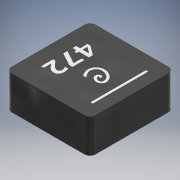
# Autodesk Inventor part: Inductor_7575
Saved by Autodesk Inventor 2018 (Build 220112000, 112)
## iProperties
Created: 2018-09-29
Part Number: Inductor_7575
Material: Steel, Carbon
Document SubType Name: Modeling
Designer: Bradley
Density: 4.9816 g/cm^3
Appearance: Fine Textured - Black
Mass: 0.85 g
Surface Area: 2.02842 cm^2
Volume: 0.170628 cm^3
Author: Bradley
Autodesk Inventor part; units mm, degrees
ref_plane "YZ Plane" through (0, 0, 0) normal (1, 0, 0) x (0, 1, 0)
ref_plane "XZ Plane" through (0, 0, 0) normal (0, 1, 0) x (-1, 0, 0)
ref_plane "XY Plane" through (0, 0, 0) normal (0, 0, 1) x (1, 0, 0)
sketch "Sketch1" plane through (0, 0, 0) normal (0, 0, 1) x (1, 0, 0)
  line L0 (3.25, -3.75) -> (-3.25, -3.75)
  line L1 (-3.75, -3.25) -> (-3.75, 3.25)
  line L2 (-3.25, 3.75) -> (3.25, 3.75)
  line L3 (3.75, 3.25) -> (3.75, -3.25)
  line L4 (3.75, -3.75) -> (-3.75, 3.75) construction
  line L5 (-3.75, -3.75) -> (3.75, 3.75) construction
  arc A0 (-3.25, 3.75) -> (-3.75, 3.25) centre (-3.25, 3.25) ccw
  arc A1 (-3.75, -3.25) -> (-3.25, -3.75) centre (-3.25, -3.25) ccw
  arc A2 (3.25, -3.75) -> (3.75, -3.25) centre (3.25, -3.25) ccw
  arc A3 (3.75, 3.25) -> (3.25, 3.75) centre (3.25, 3.25) ccw
  point P0 (0, 0)
  dimension "d0" = 7.5
  dimension "d1" = 0.5
  constraints: 12 end point, 8 point on circle, 8 point on line, 8 tangent, 4 centre point, 3 equal radius, 2 midpoint, 2 parallel, 2 perpendicular, 1 horizontal
  measures "d0" distance of L4.end L5.end
  measures "d1" radius of A0
extrude "Extrusion1" add sketch "Sketch1" along normal mid plane 3.02
sketch "Sketch2" plane through (0, 0, -1.51) normal (0, 0, -1) x (-1, 0, 0)
  line L0 (2.96, -3) -> (1.56, -3)
  line L1 (1.56, -3) -> (1.56, 3)
  line L2 (1.56, 3) -> (2.96, 3)
  line L3 (2.96, 3) -> (2.96, -3)
  line L4 (-1.56, -3) -> (-2.96, -3)
  line L5 (-2.96, -3) -> (-2.96, 3)
  line L6 (-2.96, 3) -> (-1.56, 3)
  line L7 (-1.56, 3) -> (-1.56, -3)
  line L8 (0, -3) -> (0, 3) construction
  point P0 (0, 0)
  point P1 (0, 0)
  dimension "d4" = 1.4
  dimension "d5" = 6
  dimension "d6" = 3.12
  constraints: 18 end point, 4 parallel, 4 point on line, 2 horizontal, 2 perpendicular, 1 coincident, 1 midpoint, 1 vertical, 2 other
  measures "d4" distance of L0.start L0.end
  measures "d5" distance of L2.end L0.start
  measures "d6" distance between parallel lines of L7 L1
extrude "Extrusion2" add sketch "Sketch2" along normal blind 0.08
sketch "Sketch3" plane through (0, 0, 1.51) normal (0, 0, 1) x (1, 0, 0)
  line L0 (2.75, 2.5) -> (2.5, 2.5)
  line L1 (2.5, 2.5) -> (2.5, -2.5)
  line L2 (2.5, -2.5) -> (2.75, -2.5)
  line L3 (2.75, -2.5) -> (2.75, 2.5)
  line L4 (-2.5, 2.5) -> (-2.5, -2.5) construction
  spline S0 degree 4 poles (1.3361, 0.4296) (1.5722, 0.2536) (1.6111, 0.0081) (1.8752, -0.3041) (1.3349, -0.7643) (0.9016, -0.6061) (0.6086, -0.3512) (0.6279, 0.0301) (0.8528, 0.1857) (1.2221, 0.0137) (1.0663, -0.2096) (0.9971, -0.1716) (0.8339, -0.0827) (0.9372, -0.3475) (1.124, -0.4244) (1.5104, -0.4795) (1.4218, 0.1865) (0.9203, 0.4463) (0.2397, 0.5724) (-0.0703, -0.2361) (0.2655, -0.4716) (0.366, -0.6909) (0.4591, -0.7727) knots 0 0 0 0 0 0.123761 0.174234 0.226685 0.279962 0.33014 0.377129 0.419078 0.455262 0.487036 0.514913 0.545248 0.580512 0.622872 0.674906 0.733244 0.796807 0.860625 0.919671 1 1 1 1 1
  line L5 (0.3021, -0.6347) -> (0.6161, -0.9108) construction
  arc A0 (0.3672, -0.6474) -> (0.5952, -0.8479) centre (0.698, -0.5011) ccw construction
  spline S1 degree 4 poles (1.3361, 0.4296) (1.1748, 0.5523) (0.7861, 0.8379) (-0.1178, 0.7487) (-0.2762, -0.1647) (0.0057, -0.6403) (0.1538, -0.7727) knots 0 0 0 0 0 0.46045 0.670358 1 1 1 1 1
  line L6 (-0.0024, -0.6331) -> (0.3101, -0.9124) construction
  arc A1 (0.0518, -0.6477) -> (0.2895, -0.8602) centre (0.4983, -0.3874) ccw construction
  line L7 (0.4591, -0.7727) -> (0.1538, -0.7727)
  line L8 (1.4819, -0.2272) -> (1.2942, 0.2269) construction
  arc A2 (1.4343, -0.1846) -> (1.2905, 0.1631) centre (0.7871, -0.2485) ccw construction
  line L9 (-2.1499, 0.6983) -> (-2.1499, 0.9013)
  line L10 (-2.1499, 0.9013) -> (-2.5036, 0.9013)
  line L11 (-2.5036, 0.9013) -> (-2.5036, 1.2648)
  line L12 (-2.5036, 1.2648) -> (-2.1499, 1.2648)
  line L13 (-2.1499, 1.2648) -> (-2.1499, 1.9261)
  line L14 (-2.1499, 1.9261) -> (-1.8703, 1.9261)
  line L15 (-1.8703, 1.9261) -> (-1, 1.2769)
  line L16 (-1, 1.2769) -> (-1, 0.9013)
  line L17 (-1, 0.9013) -> (-1.8801, 0.9013)
  line L18 (-1.8801, 0.9013) -> (-1.8801, 0.6983)
  line L19 (-1.8801, 0.6983) -> (-2.1499, 0.6983)
  line L20 (-1.8801, 1.2648) -> (-1.3695, 1.2648)
  line L21 (-1.3695, 1.2648) -> (-1.8801, 1.6453)
  line L22 (-1.8801, 1.6453) -> (-1.8801, 1.2648)
  line L23 (-1.2978, -0.5646) -> (-2.5, 0.076)
  line L24 (-2.5, 0.076) -> (-2.5, 0.4941)
  line L25 (-2.5, 0.4941) -> (-1.2832, -0.1756)
  line L26 (-1.2832, -0.1756) -> (-1.2832, 0.5391)
  line L27 (-1.2832, 0.5391) -> (-1, 0.5391)
  line L28 (-1, 0.5391) -> (-1, -0.5646)
  line L29 (-1, -0.5646) -> (-1.2978, -0.5646)
  line L30 (-2.5, -1.9115) -> (-2.5, -0.809)
  line L31 (-2.5, -0.809) -> (-2.2557, -0.809)
  spline S2 degree 2 poles (-2.2557, -0.809) (-2.1438, -0.9487) (-1.9469, -1.1724) (-1.8582, -1.2563) knots 0 0 0 1 2 2 2
  spline S3 degree 2 poles (-1.8582, -1.2563) (-1.7427, -1.3669) (-1.5665, -1.4654) (-1.4741, -1.4654) knots 0 0 0 1 2 2 2
  spline S4 degree 2 poles (-1.4741, -1.4654) (-1.3695, -1.4654) (-1.2577, -1.3402) (-1.2577, -1.2283) knots 0 0 0 1 2 2 2
  spline S5 degree 2 poles (-1.2577, -1.2283) (-1.2577, -1.1712) (-1.2857, -1.0691) (-1.3075, -1.0168) knots 0 0 0 1 2 2 2
  spline S6 degree 2 poles (-1.3075, -1.0168) (-1.3306, -0.9658) (-1.3793, -0.8928) (-1.3914, -0.8746) knots 0 0 0 1 2 2 2
  line L32 (-1.3914, -0.8746) -> (-1.3914, -0.8454)
  line L33 (-1.3914, -0.8454) -> (-1.0644, -0.8454)
  spline S7 degree 2 poles (-1.0644, -0.8454) (-1.034, -0.9086) (-0.9708, -1.1785) (-0.9708, -1.3037) knots 0 0 0 1 2 2 2
  spline S8 degree 2 poles (-0.9708, -1.3037) (-0.9708, -1.5711) (-1.2091, -1.8458) (-1.4242, -1.8458) knots 0 0 0 1 2 2 2
  spline S9 degree 2 poles (-1.4242, -1.8458) (-1.5567, -1.8458) (-1.812, -1.7206) (-1.9579, -1.576) knots 0 0 0 1 2 2 2
  spline S10 degree 2 poles (-1.9579, -1.576) (-2.0478, -1.4848) (-2.1876, -1.3134) (-2.2168, -1.2757) knots 0 0 0 1 2 2 2
  line L34 (-2.2168, -1.2757) -> (-2.2168, -1.9115)
  line L35 (-2.2168, -1.9115) -> (-2.5, -1.9115)
  point P0 (0, 0)
  point P1 (-2.5, 0)
  point P2 (2.5, 0)
  point P3 (1.5897, 0.1222)
  point P4 (1.6836, -0.1324)
  point P5 (1.6666, -0.392)
  point P6 (1.348, -0.657)
  point P7 (0.9064, -0.5696)
  point P8 (0.6595, -0.2864)
  point P9 (0.6874, 0.0129)
  point P10 (0.9152, 0.1153)
  point P11 (1.131, -0.0524)
  point P12 (1.0559, -0.1747)
  point P13 (0.9784, -0.1613)
  point P14 (0.8944, -0.1391)
  point P15 (0.915, -0.2539)
  point P16 (1.1067, -0.4034)
  point P17 (1.3658, -0.3897)
  point P18 (1.3881, -0.0001)
  point P19 (0.911, 0.405)
  point P20 (0.2939, 0.3734)
  point P21 (0.0837, -0.1519)
  point P22 (0.2608, -0.5163)
  point P23 (1.0376, 0.6174)
  point P24 (0.5316, 0.7174)
  point P25 (0.0302, 0.4881)
  point P26 (-0.1564, -0.1329)
  dimension "d9" = 5
  dimension "d10" = 0.25
  dimension "d11" = 2.5
  dimension "d12" = 2.5
  constraints: 18 end point, 8 midpoint, 3 centre point, 3 point on circle, 2 horizontal, 2 horizontal alignment, 2 parallel, 2 vertical, 1 perpendicular, 1 point on line, 63 other
  measures "d9" distance of L2.end L0.start
  measures "d10" distance of L0.start L0.end
  measures "d11" distance from line of L1 point (0, 0)
  measures "d12" distance from line of L4 point (0, 0)
extrude "Extrusion3" add sketch "Sketch3" along normal blind 0.01
equation "\"d12\" = d11"
body "Solid1"
